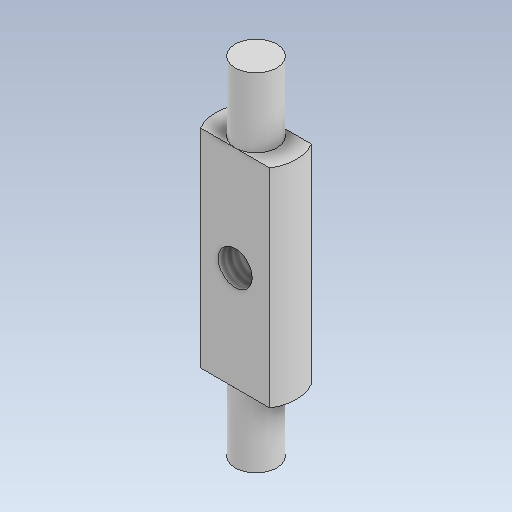
# Autodesk Inventor part: slider
Saved by Autodesk Inventor 2021 (Build 250183000, 183)
## iProperties
Created: 2020-11-23
Part Number: slider
Material: Generic
Document SubType Name: Modeling
Designer: Pysion
Density: 1 g/cm^3
Appearance: Default
Mass: 2.28438 g
Surface Area: 16.5644 cm^2
Volume: 2.28438 cm^3
Author: Pysion
Autodesk Inventor part; units mm, degrees
ref_plane "XZ Plane" through (0, 0, 0) normal (0, 1, 0) x (-1, 0, 0)
ref_plane "XY Plane" through (0, 0, 0) normal (0, 0, 1) x (1, 0, 0)
sketch "Sketch1" plane through (0, 0, 0) normal (0, 1, 0) x (-1, 0, 0)
  circle A0 centre (0, 0) radius 3
  dimension "d0" = 6
  constraints: 1 centre point, 1 coincident
  measures "d0" diameter of A0
extrude "Extrusion1" add sketch "Sketch1" along normal blind 50
ref_plane "Work Plane1" through (8, 0, 0) normal (1, 0, 0) x (0, 1, 0)
sketch "Sketch2" plane through (8, 0, 0) normal (1, 0, 0) x (0, 1, 0)
  line L0 (0, -3) -> (50, -3) projected
  line L1 (0, 3) -> (50, 3) projected
  line L2 (40, -3) -> (20, -3)
  line L3 (20, -3) -> (20, 3)
  line L4 (20, 3) -> (40, 3)
  line L5 (40, 3) -> (40, -3)
  line L6 (20, -3) -> (10, -3)
  line L7 (10, -3) -> (10, 3)
  line L8 (10, 3) -> (20, 3)
  line L9 (20, 3) -> (20, -3)
  line L10 (0, -3) -> (0, 3) projected
  line L11 (50, -3) -> (50, 3) projected
  point P0 (0, 0)
  point P1 (20, -3)
  point P2 (20, 3)
  point P3 (10, 3)
  point P4 (10, -3)
  point P5 (40, 3)
  point P6 (20, -3)
  dimension "d4" = 20
  dimension "d5" = 10
  dimension "d7" = 10
  dimension "d19" = 30
  constraints: 16 end point, 4 parallel, 4 point on line, 2 horizontal, 2 perpendicular
  measures "d4" distance of L3.end L4.end
  measures "d5" distance of L7.end L8.end
  measures "d7" distance between parallel lines of L10 L7
  measures "d19" distance between parallel lines of L5 L7
extrude "Extrusion2" add sketch "Sketch2" against normal blind 14 contours L7 L1 L3 L0 | L3 L1 L5 L0
sketch "Sketch6" plane through (8, 10, -3) normal (0, 0, -1) x (-1, 0, 0)
  circle A0 centre (8.5023, 25) radius 3
  circle A1 centre (8.5023, 5) radius 3
  line L0 (8, 30) -> (14, 30) projected
  line L1 (8, 0) -> (14, 0) projected
  point P0 (8, -10)
  dimension "d36" = 6
  dimension "d37" = 6
  dimension "d38" = 0
  dimension "d39" = 5
  dimension "d40" = 5
  constraints: 2 centre point
  measures "d36" diameter of A0
  measures "d37" diameter of A1
  measures "d38" horizontal distance of A1.centre A0.centre
  measures "d39" distance from line of L0 A0.centre
  measures "d40" distance from line of L1 A1.centre
extrude "Extrusion5" cut sketch "Sketch6" against normal blind 3
sketch "Sketch7" plane through (8, 10, -3) normal (0, 0, -1) x (-1, 0, 0)
  line L0 (14, 30) -> (14, 0) projected
  line L1 (8, 30) -> (14, 30) projected
  point P0 (8, -10)
  point P1 (8, 15)
  dimension "d43" = 6
  dimension "d44" = 15
  measures "d43" distance from line of L0 point (8, 15)
  measures "d44" distance from line of L1 point (8, 15)
hole "Hole2" at (0, 25, -3) direction (0, 0, 1) diameter 4.917 end through all thread size "M6x1" class "6H" standard "ISO Metric profile"
sketch "Sketch9" plane through (-6, 40, -3) normal (0, 1, 0) x (1, 0, 0)
  circle A0 centre (6, -3) radius 5.831
  circle A1 centre (6, -3) radius 3 projected
  circle A2 centre (6, -3) radius 10
  dimension "d54" = 11.662
  dimension "d55" = 20
  constraints: 2 centre point, 1 coincident, 1 concentric
  measures "d54" diameter of A0
  measures "d55" diameter of A2
extrude "Extrusion7" cut sketch "Sketch9" against normal blind 40 contours A2
body "Solid1"
